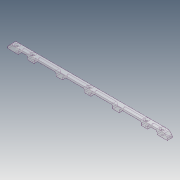
# Autodesk Inventor part: J005229
Saved by Autodesk Inventor 2015 SP1 (Build 190203100, 203)
## iProperties
Created: 2015-05-20
Material: ACRYLIC, CLEAR
Vendor: HHMI: JRC - ID&F
Document SubType Name: Modeling
Designer: ARNOLDJ
Density: 0.66 g/cm^3
Appearance: Polycarbonate (Clear)
Description: MBS TROUGH RAIL
Part Number: J005229
Project: P-201804
RuleStatus: InUse
AfterDocSave0: file://Part Number Cleaner
LAB/DEPT: SVOBODA (LAB)
REQUESTING SCIENTIST: SOFRONIEW, NICK
SURFACE ROUGHNESS: N/A
DESIGN DEPARTMENT: HHMI: JRC - ID&F
SPECIAL FINISH: NONE
ALTERED ITEM PART NUMBER: N/A
ALTERED ITEM VENDOR: N/A
ALTERED ITEM DESCRIPTION: N/A
Author: ARNOLDJ
Revision Number: -
Autodesk Inventor part; units mm, degrees
ref_plane "YZ Plane" through (0, 0, 0) normal (1, 0, 0) x (0, 1, 0)
ref_plane "XY Plane" through (0, 0, 0) normal (0, 0, 1) x (1, 0, 0)
sketch "Sketch1" plane through (0, 0, 0) normal (0, 0, 1) x (1, 0, 0)
  line L0 (0, 7.5565) -> (0, -7.5565) projected
  line L1 (-224.4725, 0) -> (224.4725, 0) projected
  line L2 (160.3375, -5.3975) -> (-160.3375, -5.3975)
  line L3 (-160.3375, -5.3975) -> (-160.3375, 5.3975)
  line L4 (-160.3375, 5.3975) -> (160.3375, 5.3975)
  line L5 (160.3375, 5.3975) -> (160.3375, -5.3975)
  line L6 (160.3375, -5.3975) -> (-160.3375, 5.3975) construction
  line L7 (-160.3375, -5.3975) -> (160.3375, 5.3975) construction
  point P0 (0, 0)
  dimension "d0" = 320.675
  dimension "d1" = 10.795
  constraints: 12 end point, 2 midpoint, 2 parallel, 1 horizontal, 1 perpendicular
  measures "d0" distance of L3.end L4.end
  measures "d1" distance of L2.end L3.end
extrude "Extrusion1" add sketch "Sketch1" along normal mid plane 9.525
sketch "Sketch2" plane through (0, 0, 0) normal (0, 0, 1) x (1, 0, 0)
  line L0 (-160.3375, 5.3975) -> (-160.3375, -5.3975) projected
  line L1 (-160.3375, -5.3975) -> (160.3375, -5.3975) projected
  line L2 (-160.3375, -5.3975) -> (160.3375, -5.3975) projected
  line L3 (160.3375, -5.3975) -> (160.3375, 5.3975) projected
  line L4 (160.3375, 5.3975) -> (-160.3375, 5.3975) projected
  line L5 (-160.3375, 5.3975) -> (-160.3375, -5.3975) projected
  line L6 (160.3375, -5.3975) -> (160.3375, 5.3975) projected
  line L7 (0, 7.5565) -> (0, -7.5565) projected
  line L8 (-139.7, -5.3975) -> (-120.65, -5.3975)
  line L9 (-120.65, -5.3975) -> (-120.65, 1.5875)
  line L10 (-120.65, 1.5875) -> (-139.7, 1.5875)
  line L11 (-139.7, 1.5875) -> (-139.7, -5.3975)
  line L12 (-107.95, -5.3975) -> (-63.5, -5.3975)
  line L13 (-63.5, -5.3975) -> (-63.5, 1.5875)
  line L14 (-63.5, 1.5875) -> (-107.95, 1.5875)
  line L15 (-107.95, 1.5875) -> (-107.95, -5.3975)
  line L16 (160.3375, 5.3975) -> (-160.3375, 5.3975) construction
  line L17 (-112.2997, -5.3975) -> (-116.3003, -5.3975) construction
  line L18 (-116.3003, -5.3975) -> (-116.3003, 5.3975) construction
  line L19 (-116.3003, 5.3975) -> (-112.2997, 5.3975) construction
  line L20 (-112.2997, 5.3975) -> (-112.2997, -5.3975) construction
  line L21 (-112.2997, -5.3975) -> (-116.3003, 5.3975) construction
  line L22 (-116.3003, -5.3975) -> (-112.2997, 5.3975) construction
  line L23 (-144.0497, -5.3975) -> (-148.0502, -5.3975) construction
  line L24 (-148.0502, -5.3975) -> (-148.0502, 5.3975) construction
  line L25 (-148.0502, 5.3975) -> (-144.0497, 5.3975) construction
  line L26 (-144.0497, 5.3975) -> (-144.0497, -5.3975) construction
  line L27 (-144.0497, -5.3975) -> (-148.0502, 5.3975) construction
  line L28 (-148.0502, -5.3975) -> (-144.0497, 5.3975) construction
  line L29 (2.0003, -5.3975) -> (-2.0002, -5.3975) construction
  line L30 (-2.0002, -5.3975) -> (-2.0003, 5.3975) construction
  line L31 (-2.0003, 5.3975) -> (2.0002, 5.3975) construction
  line L32 (2.0002, 5.3975) -> (2.0003, -5.3975) construction
  line L33 (2.0003, -5.3975) -> (-2.0003, 5.3975) construction
  line L34 (-2.0002, -5.3975) -> (2.0002, 5.3975) construction
  line L35 (116.3003, -5.3975) -> (112.2997, -5.3975) construction
  line L36 (112.2997, -5.3975) -> (112.2997, 5.3975) construction
  line L37 (112.2997, 5.3975) -> (116.3003, 5.3975) construction
  line L38 (116.3003, 5.3975) -> (116.3003, -5.3975) construction
  line L39 (116.3003, -5.3975) -> (112.2997, 5.3975) construction
  line L40 (112.2997, -5.3975) -> (116.3003, 5.3975) construction
  line L41 (148.0503, -5.3975) -> (144.0498, -5.3975) construction
  line L42 (144.0498, -5.3975) -> (144.0498, 5.3975) construction
  line L43 (144.0498, 5.3975) -> (148.0503, 5.3975) construction
  line L44 (148.0503, 5.3975) -> (148.0503, -5.3975) construction
  line L45 (148.0503, -5.3975) -> (144.0498, 5.3975) construction
  line L46 (144.0498, -5.3975) -> (148.0503, 5.3975) construction
  line L47 (-50.8, -5.3975) -> (-6.35, -5.3975)
  line L48 (-6.35, -5.3975) -> (-6.35, 1.5875)
  line L49 (-6.35, 1.5875) -> (-50.8, 1.5875)
  line L50 (-50.8, 1.5875) -> (-50.8, -5.3975)
  point P0 (0, 0)
  point P1 (-114.3, 0)
  point P2 (-146.05, 0)
  point P3 (114.3, 0)
  point P4 (146.05, 0)
  dimension "d4" = 320.675
  dimension "d5" = 4.0005
  dimension "d6" = 114.3
  dimension "d7" = 4.0005
  dimension "d8" = 31.75
  dimension "d9" = 4.0005
  dimension "d10" = 4.0005
  dimension "d11" = 114.3
  dimension "d12" = 4.0005
  dimension "d13" = 31.75
  dimension "d14" = 6.985
  dimension "d15" = 6.35
  dimension "d16" = 6.35
  dimension "d17" = 6.35
  dimension "d19" = 6.985
  dimension "d20" = 6.35
  dimension "d21" = 19.05
  dimension "d22" = 12.7
  constraints: 84 end point, 16 parallel, 10 midpoint, 9 point on line, 8 horizontal, 8 perpendicular, 1 collinear
  measures "d4" distance of L3.end L4.end
  measures "d5" distance of L18.end L19.end
  measures "d6" distance from line of L7 point (-114.3, 0)
  measures "d7" distance of L24.end L25.end
  measures "d8" distance of point (-146.05, 0) point (-114.3, 0)
  measures "d9" distance of L30.end L31.end
  measures "d10" distance of L36.end L37.end
  measures "d11" distance of point (0, 0) point (114.3, 0)
  measures "d12" distance of L42.end L43.end
  measures "d13" distance of point (146.05, 0) point (114.3, 0)
  measures "d14" distance of L10.end L8.start
  measures "d15" distance from line of L11 point (-146.05, 0)
  measures "d16" distance from line of L9 point (-114.3, 0)
  measures "d17" distance from line of L15 point (-114.3, 0)
  measures "d19" distance of L49.end L47.start
  measures "d20" distance from line of L48 point (0, 0)
  measures "d21" distance of L9.end L10.end
  measures "d22" distance between parallel lines of L50 L13
extrude "Extrusion2" cut sketch "Sketch2" along normal up to surface (9.525 mm away) from surface at -4.7625 contours L11 L10 L9 L1 | L1 L50 L49 L48 | L15 L14 L13 L1
chamfer "Chamfer1" distance 6.35 angle 45 1 edges at (-160.3375, 5.3975, 0)
mirror "Mirror1" about plane through (0, 0, 0) normal (1, 0, 0) of "Extrusion2"
fillet "Fillet1" radius 3.175 12 edges at (-139.7, 1.5875, 0) (-120.65, 1.5875, 0) (-107.95, 1.5875, 0) (-63.5, 1.5875, 0) (-50.8, 1.5875, 0) (-6.35, 1.5875, 0) (6.35, 1.5875, 0) (50.8, 1.5875, 0) (63.5, 1.5875, 0) (107.95, 1.5875, 0) (120.65, 1.5875, 0) (139.7, 1.5875, 0)
chamfer "Chamfer2" distance 6.35 angle 45 1 edges at (160.3375, 5.3975, 0)
fillet "Fillet2" radius 3.175 4 edges at (153.9875, 5.3975, 0) (160.3375, -0.9525, 0) (-160.3375, -0.9525, 0) (-153.9875, 5.3975, 0)
ref_plane "Work Plane1" through (0, 5.4102, 0) normal (0, 1, 0) x (-1, 0, 0)
sketch "Sketch3" plane through (0, 5.4102, 0) normal (0, 1, 0) x (-1, 0, 0)
  line L0 (0, -204.47) -> (0, 204.47) projected
  line L1 (-204.47, 0) -> (204.47, 0) projected
  point P0 (0, 0)
  point P1 (114.3, 0)
  point P2 (146.05, 0)
  point P3 (0, 0)
  point P4 (-146.05, 0)
  point P5 (-114.3, 0)
  dimension "d34" = 31.75
  dimension "d35" = 114.3
  dimension "d36" = 31.75
  dimension "d37" = 114.3
  constraints: 4 point on line, 1 coincident
  measures "d34" distance of point (-146.05, 0) point (-114.3, 0)
  measures "d35" distance from line of L0 point (-114.3, 0)
  measures "d36" distance of point (114.3, 0) point (146.05, 0)
  measures "d37" distance of point (0, 0) point (114.3, 0)
hole "Hole1" at (-114.3, 5.4102, 0) at (-146.05, 5.4102, 0) at (0, 5.4102, 0) at (146.05, 5.4102, 0) at (114.3, 5.4102, 0) direction (0, -1, 0) diameter 4.8006 end through all countersink diameter 9.398 countersink angle 90 clearance for "Flat Head Machine Screw" size "M4" standard "Ansi Metric M Profile"
body "Solid1"
